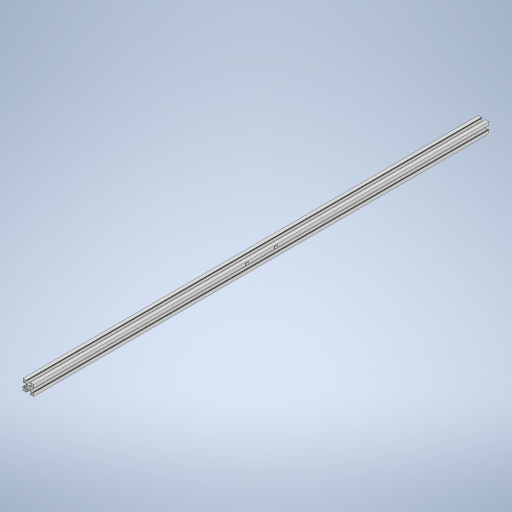
# Autodesk Inventor part: T slot beam 20mm
Saved by Autodesk Inventor 2023.5 (Build 275446000, 446)
## iProperties
Created: 2024-07-24
Part Number: T slot beam 20mm
Material: Generic
Document SubType Name: Modeling
Designer: Big Sean T
Density: 1 g/cm^3
Appearance: Default
Author: Big Sean T
Autodesk Inventor part; units mm, degrees
ref_plane "YZ Plane" through (0, 0, 0) normal (1, 0, 0) x (0, 1, 0)
ref_plane "XZ Plane" through (0, 0, 0) normal (0, 1, 0) x (-1, 0, 0)
ref_plane "XY Plane" through (0, 0, 0) normal (0, 0, 1) x (1, 0, 0)
sketch "Sketch1" plane through (0, 0, 0) normal (0, 0, 1) x (1, 0, 0)
  line L0 (0, 0) -> (6.146, 0)
  line L1 (6.4, 0.254) -> (6.4, 0.5)
  line L2 (6.4, 0.5) -> (6.646, 0.5)
  line L3 (6.9, 0.754) -> (6.9, 1.546)
  line L4 (0, 0) -> (0, 6.146)
  line L5 (0.254, 6.4) -> (0.5, 6.4)
  line L6 (0.5, 6.4) -> (0.5, 6.646)
  line L7 (0.754, 6.9) -> (1.5449, 6.9)
  line L8 (1.7989, 6.646) -> (1.7989, 4.8147)
  line L9 (6.646, 1.8) -> (4.754, 1.8)
  line L10 (20, 0) -> (20, 6.146)
  line L11 (19.746, 6.4) -> (19.5, 6.4)
  line L12 (19.5, 6.4) -> (19.5, 6.646)
  line L13 (19.246, 6.9) -> (18.4551, 6.9)
  line L14 (18.2011, 6.646) -> (18.2011, 4.8147)
  line L15 (20, 0) -> (13.854, 0)
  line L16 (13.6, 0.254) -> (13.6, 0.5)
  circle A0 centre (10, 10) radius 2.5
  line L17 (20, 20) -> (13.854, 20)
  line L18 (20, 20) -> (20, 13.854)
  line L19 (19.746, 13.6) -> (19.5, 13.6)
  line L20 (19.5, 13.6) -> (19.5, 13.354)
  line L21 (19.246, 13.1) -> (18.454, 13.1)
  line L22 (13.6, 19.746) -> (13.6, 19.5)
  line L23 (13.6, 19.5) -> (13.354, 19.5)
  line L24 (13.1, 19.246) -> (13.1, 18.454)
  line L25 (13.354, 18.2) -> (15.246, 18.2)
  line L26 (0, 20) -> (6.146, 20)
  line L27 (6.4, 19.746) -> (6.4, 19.5)
  line L28 (6.4, 19.5) -> (6.646, 19.5)
  line L29 (6.9, 19.246) -> (6.9, 18.454)
  line L30 (6.646, 18.2) -> (4.754, 18.2)
  line L31 (0, 20) -> (0, 13.854)
  line L32 (0.254, 13.6) -> (0.5, 13.6)
  line L33 (0.5, 13.6) -> (0.5, 13.354)
  line L34 (0.754, 13.1) -> (1.546, 13.1)
  line L35 (1.8, 13.354) -> (1.8, 15.246)
  line L36 (3.4393, 15.5) -> (2.054, 15.5)
  line L37 (4.5, 16.5607) -> (4.5, 17.946)
  line L38 (16.5, 4.5607) -> (17.9471, 4.5607)
  line L39 (13.6, 0.5) -> (13.354, 0.5)
  line L40 (13.1, 0.754) -> (13.1, 1.546)
  line L41 (13.354, 1.8) -> (15.246, 1.8)
  line L42 (15.5, 2.054) -> (15.5, 3.4393)
  line L43 (15.5, 16.5607) -> (15.5, 17.946)
  line L44 (16.5, 15.4393) -> (17.946, 15.4393)
  line L45 (4.5, 3.4393) -> (4.5, 2.054)
  line L46 (3.5, 4.5607) -> (2.0529, 4.5607)
  line L47 (6.1, 7.6867) -> (6.1, 12.3133)
  line L48 (3.5, 4.5607) -> (5.728, 6.7887)
  line L49 (3.4393, 15.5) -> (5.728, 13.2113)
  line L50 (7.6867, 13.9) -> (12.3133, 13.9)
  line L51 (6.7887, 14.272) -> (4.5, 16.5607)
  line L52 (13.2113, 14.272) -> (15.5, 16.5607)
  line L53 (13.9, 12.3133) -> (13.9, 7.6867)
  line L54 (14.272, 6.7887) -> (16.5, 4.5607)
  line L55 (14.272, 13.2113) -> (16.5, 15.4393)
  line L56 (7.6867, 6.1) -> (12.3133, 6.1)
  line L57 (6.7887, 5.728) -> (4.5, 3.4393)
  line L58 (13.2113, 5.728) -> (15.5, 3.4393)
  arc A1 (6.9, 19.246) -> (6.646, 19.5) centre (6.646, 19.246) ccw
  arc A2 (6.4, 19.746) -> (6.146, 20) centre (6.146, 19.746) ccw
  arc A3 (6.646, 18.2) -> (6.9, 18.454) centre (6.646, 18.454) ccw
  arc A4 (4.754, 18.2) -> (4.5, 17.946) centre (4.754, 17.946) ccw
  arc A5 (13.1, 18.454) -> (13.354, 18.2) centre (13.354, 18.454) ccw
  arc A6 (13.354, 19.5) -> (13.1, 19.246) centre (13.354, 19.246) ccw
  arc A7 (13.854, 20) -> (13.6, 19.746) centre (13.854, 19.746) ccw
  arc A8 (15.5, 17.946) -> (15.246, 18.2) centre (15.246, 17.946) ccw
  arc A9 (2.054, 15.5) -> (1.8, 15.246) centre (2.054, 15.246) ccw
  arc A10 (0.5, 13.354) -> (0.754, 13.1) centre (0.754, 13.354) ccw
  arc A11 (0, 13.854) -> (0.254, 13.6) centre (0.254, 13.854) ccw
  arc A12 (1.546, 13.1) -> (1.8, 13.354) centre (1.546, 13.354) ccw
  arc A13 (0.254, 6.4) -> (0, 6.146) centre (0.254, 6.146) ccw
  arc A14 (0.754, 6.9) -> (0.5, 6.646) centre (0.754, 6.646) ccw
  arc A15 (1.7989, 6.646) -> (1.5449, 6.9) centre (1.5449, 6.646) ccw
  arc A16 (1.7989, 4.8147) -> (2.0529, 4.5607) centre (2.0529, 4.8147) ccw
  arc A17 (19.746, 13.6) -> (20, 13.854) centre (19.746, 13.854) ccw
  arc A18 (19.246, 13.1) -> (19.5, 13.354) centre (19.246, 13.354) ccw
  arc A19 (18.2, 13.354) -> (18.454, 13.1) centre (18.454, 13.354) ccw
  line L59 (18.2, 13.354) -> (18.2, 15.1853)
  arc A20 (18.2, 15.1853) -> (17.946, 15.4393) centre (17.946, 15.1853) ccw
  arc A21 (20, 6.146) -> (19.746, 6.4) centre (19.746, 6.146) ccw
  arc A22 (19.5, 6.646) -> (19.246, 6.9) centre (19.246, 6.646) ccw
  arc A23 (18.4551, 6.9) -> (18.2011, 6.646) centre (18.4551, 6.646) ccw
  arc A24 (17.9471, 4.5607) -> (18.2011, 4.8147) centre (17.9471, 4.8147) ccw
  arc A25 (13.6, 0.254) -> (13.854, 0) centre (13.854, 0.254) ccw
  arc A26 (13.1, 0.754) -> (13.354, 0.5) centre (13.354, 0.754) ccw
  arc A27 (13.354, 1.8) -> (13.1, 1.546) centre (13.354, 1.546) ccw
  arc A28 (15.246, 1.8) -> (15.5, 2.054) centre (15.246, 2.054) ccw
  arc A29 (6.146, 0) -> (6.4, 0.254) centre (6.146, 0.254) ccw
  arc A30 (6.646, 0.5) -> (6.9, 0.754) centre (6.646, 0.754) ccw
  arc A31 (6.9, 1.546) -> (6.646, 1.8) centre (6.646, 1.546) ccw
  arc A32 (4.5, 2.054) -> (4.754, 1.8) centre (4.754, 2.054) ccw
  arc A33 (6.7887, 14.272) -> (7.6867, 13.9) centre (7.6867, 15.17) ccw
  arc A34 (12.3133, 13.9) -> (13.2113, 14.272) centre (12.3133, 15.17) ccw
  arc A35 (6.1, 12.3133) -> (5.728, 13.2113) centre (4.83, 12.3133) ccw
  arc A36 (5.728, 6.7887) -> (6.1, 7.6867) centre (4.83, 7.6867) ccw
  arc A37 (7.6867, 6.1) -> (6.7887, 5.728) centre (7.6867, 4.83) ccw
  arc A38 (13.2113, 5.728) -> (12.3133, 6.1) centre (12.3133, 4.83) ccw
  arc A39 (13.9, 7.6867) -> (14.272, 6.7887) centre (15.17, 7.6867) ccw
  arc A40 (14.272, 13.2113) -> (13.9, 12.3133) centre (15.17, 12.3133) ccw
  point P0 (20, 6.4)
  point P1 (19.5, 6.9)
  point P2 (18.2011, 6.9)
  dimension "d59" = 1.27
  constraints: 120 end point, 80 point on circle, 79 tangent, 41 centre point, 37 equal radius, 32 perpendicular, 12 point on line, 6 horizontal, 2 vertical, 1 collinear, 1 parallel
  measures "d59" radius of A33
extrude "Extrusion1" add sketch "Sketch1" along normal blind 862.076
sketch "Sketch5" plane through (0, 0, 0) normal (-1, 0, 0) x (0, 0, 1)
  line L0 (0, 5.728) -> (862.076, 5.728) projected
  line L1 (0, 0) -> (0, 5.728)
  line L2 (0, 5.728) -> (6, 5.728)
  line L3 (6, 5.728) -> (6, 0.5)
  line L4 (0, 0.5) -> (862.076, 0.5) projected
  line L5 (0, 0.5) -> (6, 0.5)
  dimension "d69" = 6
  constraints: 8 end point, 2 perpendicular, 2 point on line, 1 collinear
  measures "d69" distance of L0.start L2.end
extrude "Extrusion2" add sketch "Sketch5" along normal blind 0.635
sketch "Sketch6" plane through (0, 0, 0) normal (-1, 0, 0) x (0, 0, 1)
  line L0 (0, 0) -> (431.038, 0)
  line L1 (0, 20) -> (862.076, 20) projected
  line L2 (431.038, 0) -> (428.038, 0)
  line L3 (0, 0) -> (862.076, 0) projected
  line L4 (428.038, 0) -> (428.038, 6.146)
  line L5 (0, 6.146) -> (862.076, 6.146) projected
  line L6 (428.038, 6.146) -> (434.0378, 6.1)
  line L7 (0, 6.1) -> (862.076, 6.1) projected
  line L8 (434.0378, 6.1) -> (433.9911, 0)
  line L9 (433.9911, 0) -> (431.038, 0)
  line L10 (862.076, 0) -> (862.076, 6.1)
  line L11 (862.076, 6.146) -> (862.076, 6.4) projected
  line L12 (862.076, 6.146) -> (856.0762, 6.1)
  line L13 (856.0762, 6.1) -> (856.0762, 0)
  line L14 (862.076, 0) -> (856.0762, 0)
  line L15 (0, 0.254) -> (862.076, 0.254) projected
  point P0 (856.0762, 0.254)
  dimension "d72" = 3
  dimension "d73" = 6
  dimension "d74" = 6
  constraints: 20 end point, 7 point on line, 3 perpendicular, 2 parallel, 1 vertical
  measures "d72" distance of L0.end L2.end
  measures "d73" distance of L4.end L6.end
  measures "d74" distance of L5.end L12.end
extrude "Extrusion3" add sketch "Sketch6" along normal blind 0.635 contours L4 L15 L8 L3 L0 | L4 L7 L8 L15 | L4 L6 L7 | L13 L7 L10 L15
sketch "Sketch7" plane through (20, 6.146, 862.076) normal (1, 0, 0) x (0, 0, -1)
  line L0 (862.076, 12.308) -> (0, 12.308) projected
  line L1 (0, 12.308) -> (431.038, 12.308)
  line L2 (862.076, 6.1673) -> (0, 6.1673) projected
  line L3 (431.038, 12.308) -> (458.538, 12.308)
  line L4 (431.038, 12.308) -> (403.538, 12.308)
  line L5 (403.538, 12.308) -> (403.538, 8.126)
  line L6 (862.076, 8.126) -> (0, 8.126) projected
  line L7 (403.538, 12.308) -> (400.538, 12.308)
  line L8 (400.538, 12.308) -> (406.538, 12.308)
  line L9 (406.538, 12.308) -> (406.538, 8.126)
  line L10 (406.538, 8.126) -> (400.538, 8.126)
  line L11 (400.538, 8.126) -> (400.538, 12.308)
  line L12 (458.538, 12.308) -> (461.538, 12.308)
  line L13 (461.538, 12.308) -> (461.538, 8.126)
  line L14 (461.538, 8.126) -> (455.538, 8.126)
  line L15 (455.538, 8.126) -> (455.538, 12.308)
  line L16 (458.538, 12.308) -> (455.538, 12.308)
  point P0 (862.076, -6.146)
  point P1 (406.538, 8.126)
  dimension "d77" = 27.5
  dimension "d78" = 27.5
  dimension "d79" = 3
  dimension "d80" = 6
  dimension "d81" = 3
  dimension "d82" = 6
  constraints: 28 end point, 9 point on line, 6 perpendicular, 1 collinear, 1 parallel
  measures "d77" distance of L1.end L3.end
  measures "d78" distance of L1.end L4.end
  measures "d79" distance of L4.end L7.end
  measures "d80" distance of L7.end L8.end
  measures "d81" distance of L3.end L12.end
  measures "d82" distance of L13.end L14.end
extrude "Extrusion4" add sketch "Sketch7" along normal blind 0.635 contours L13 L6 L15 L0 | L6 L5 L0 L9 | L6 L11 L0 L5
sketch "Sketch8" plane through (20.635, 6.146, 862.076) normal (1, 0, 0) x (0, 0, -1)
  point P0 (862.076, -6.146)
body "Solid1"
